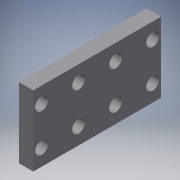
# Autodesk Inventor part: USB Wärmeableiter 2
Saved by Autodesk Inventor 2017 (Build 210142000, 142)
## iProperties
Part Number: USB Wärmeableiter 2
Material: Generisch
Document SubType Name: Modeling
Designer: David Merges
Density: 1 g/cm^3
Appearance: Vorgabe
Author: David Merges
Autodesk Inventor part; units mm, degrees
ref_plane "YZ Plane" through (0, 0, 0) normal (1, 0, 0) x (0, 1, 0)
ref_plane "XZ Plane" through (0, 0, 0) normal (0, 1, 0) x (-1, 0, 0)
ref_plane "XY Plane" through (0, 0, 0) normal (0, 0, 1) x (1, 0, 0)
sketch "Skizze1" plane through (0, 0, 0) normal (0, 0, 1) x (1, 0, 0)
  line L0 (-1.5, 13.45) -> (1.5, 13.45)
  line L1 (1.5, 13.45) -> (1.5, -13.45)
  line L2 (1.5, -13.45) -> (-1.5, -13.45)
  line L3 (-1.5, -13.45) -> (-1.5, 13.45)
  line L4 (-1.5, -13.45) -> (1.5, 13.45) construction
  point P0 (0, 0)
  point P1 (0, 0)
  dimension "d0" = 3
  dimension "d1" = 26.9
  constraints: 10 end point, 2 parallel, 1 coincident, 1 horizontal, 1 midpoint, 1 perpendicular
  measures "d0" distance of L1.end L2.end
  measures "d1" distance of L0.end L1.end
extrude "Extrusion1" add sketch "Skizze1" along normal blind 14.8
sketch "Skizze2" plane through (-1.5, -13.45, 0) normal (-1, 0, 0) x (0, 0, 1)
  circle A0 centre (11.5, 25.15) radius 1.0065 projected
  circle A1 centre (3.5, 25.15) radius 1.0065 projected
  circle A2 centre (11.5, 17.35) radius 1.0065 projected
  circle A3 centre (3.5, 17.35) radius 1.0065 projected
  circle A4 centre (3.5, 9.55) radius 1.0065 projected
  circle A5 centre (11.5, 9.55) radius 1.0065 projected
  circle A6 centre (11.5, 1.75) radius 1.0065 projected
  circle A7 centre (3.5, 1.75) radius 1.0065 projected
  point P0 (0, 13.45)
hole "Bohrung1" at (-1.5, 11.7, 11.5) at (-1.5, 11.7, 3.5) at (-1.5, 3.9, 3.5) at (-1.5, 3.9, 11.5) at (-1.5, -3.9, 11.5) at (-1.5, -3.9, 3.5) at (-1.5, -11.7, 3.5) at (-1.5, -11.7, 11.5) direction (1, 0, 0) diameter 2.7 end through all
